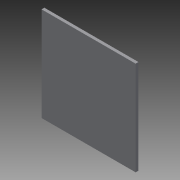
# Autodesk Inventor part: fai20_sikiita
Saved by Autodesk Inventor 2013 (Build 170138000, 138)
## iProperties
Created: 2014-04-21
Part Number: fai20_sikiita
Material: 一般
Document SubType Name: Modeling
Designer: andou
Density: 1 g/cm^3
Author: andou
Autodesk Inventor part; units mm, degrees
ref_plane "YZ Plane" through (0, 0, 0) normal (1, 0, 0) x (0, 1, 0)
ref_plane "XZ Plane" through (0, 0, 0) normal (0, 1, 0) x (-1, 0, 0)
ref_plane "XY Plane" through (0, 0, 0) normal (0, 0, 1) x (1, 0, 0)
sketch "スケッチ1" plane through (0, 0, 0) normal (0, 1, 0) x (-1, 0, 0)
  line L0 (-50, 50) -> (50, 50)
  line L1 (50, 50) -> (50, -50)
  line L2 (50, -50) -> (-50, -50)
  line L3 (-50, -50) -> (-50, 50)
  point P0 (0, 0)
  dimension "d0" = 100
  dimension "d2" = 100
  dimension "d3" = 50
  dimension "d4" = 50
  constraints: 8 end point, 2 parallel, 1 horizontal, 1 perpendicular
  measures "d0" distance of L0.start L0.end
  measures "d2" distance of L2.end L0.start
  measures "d3" distance from line of L0 point (0, 0)
  measures "d4" distance from line of L3 point (0, 0)
extrude "押し出し1" add sketch "スケッチ1" along normal blind 2
sketch "スケッチ2" plane through (0, 2, 0) normal (0, 1, 0) x (1, 0, 0)
  line L0 (-50, -50) -> (50, -50) projected
  line L1 (50, -50) -> (50, 50) projected
  line L2 (50, 50) -> (-50, 50) projected
  line L3 (-50, 50) -> (-50, -50) projected
  circle A0 centre (-38, -38) radius 10
  circle A1 centre (-13, -38) radius 10
  circle A2 centre (12, -38) radius 10
  circle A3 centre (-38, -13) radius 10
  circle A4 centre (-13, -13) radius 10
  circle A5 centre (12, -13) radius 10
  circle A6 centre (-38, 12) radius 10
  circle A7 centre (-13, 12) radius 10
  circle A8 centre (12, 12) radius 10
  circle A9 centre (37, -38) radius 10
  circle A10 centre (37, -13) radius 10
  circle A11 centre (37, 12) radius 10
  circle A12 centre (37, 37) radius 10
  circle A13 centre (12, 37) radius 10
  circle A14 centre (-13, 37) radius 10
  circle A15 centre (-38, 37) radius 10
  point P0 (0, 0)
  dimension "d7" = 20
  dimension "d9" = 25
  dimension "d10" = 25
  dimension "d11" = 12
  dimension "d12" = 12
  dimension "d13" = 12
  dimension "d14" = 12
  dimension "d15" = 25
  dimension "d16" = 25
  dimension "d17" = 12
  dimension "d18" = 25
  dimension "d19" = 25
  dimension "d20" = 25
  dimension "d21" = 25
  dimension "d22" = 25
  dimension "d23" = 25
  dimension "d24" = 25
  dimension "d25" = 25
  dimension "d26" = 12
  dimension "d27" = 25
  dimension "d28" = 12
  dimension "d29" = 25
  dimension "d30" = 25
  dimension "d31" = 25
  dimension "d32" = 25
  dimension "d33" = 25
  dimension "d34" = 25
  dimension "d35" = 25
  dimension "d36" = 25
  dimension "d37" = 25
  dimension "d38" = 25
  dimension "d39" = 25
  dimension "d40" = 12
  constraints: 16 centre point, 15 equal radius
  measures "d7" diameter of A0
  measures "d9" distance of A1.centre A0.centre
  measures "d10" distance of A2.centre A1.centre
  measures "d11" distance from line of A0.centre L0
  measures "d12" distance from line of L3 A0.centre
  measures "d13" distance from line of L0 A1.centre
  measures "d14" distance from line of A2.centre L0
  measures "d15" distance of A4.centre A3.centre
  measures "d16" distance of A5.centre A4.centre
  measures "d17" distance from line of L3 A3.centre
  measures "d18" distance of A3.centre A0.centre
  measures "d19" distance of A6.centre A3.centre
  measures "d20" distance of A1.centre A4.centre
  measures "d21" distance of A2.centre A5.centre
  measures "d22" distance of A8.centre A5.centre
  measures "d23" distance of A7.centre A4.centre
  measures "d24" distance of A7.centre A6.centre
  measures "d25" distance of A8.centre A7.centre
  measures "d26" distance from line of L3 A6.centre
  measures "d27" distance of A9.centre A2.centre
  measures "d28" distance from line of L0 A9.centre
  measures "d29" distance of A10.centre A9.centre
  measures "d30" distance of A10.centre A11.centre
  measures "d31" distance of A11.centre A12.centre
  measures "d32" distance of A8.centre A11.centre
  measures "d33" distance of A5.centre A10.centre
  measures "d34" distance of A13.centre A12.centre
  measures "d35" distance of A14.centre A13.centre
  measures "d36" distance of A15.centre A14.centre
  measures "d37" distance of A15.centre A6.centre
  measures "d38" distance of A14.centre A7.centre
  measures "d39" distance of A13.centre A8.centre
  measures "d40" distance from line of L3 A15.centre
extrude "押し出し2" add sketch "スケッチ2" along normal blind 1
